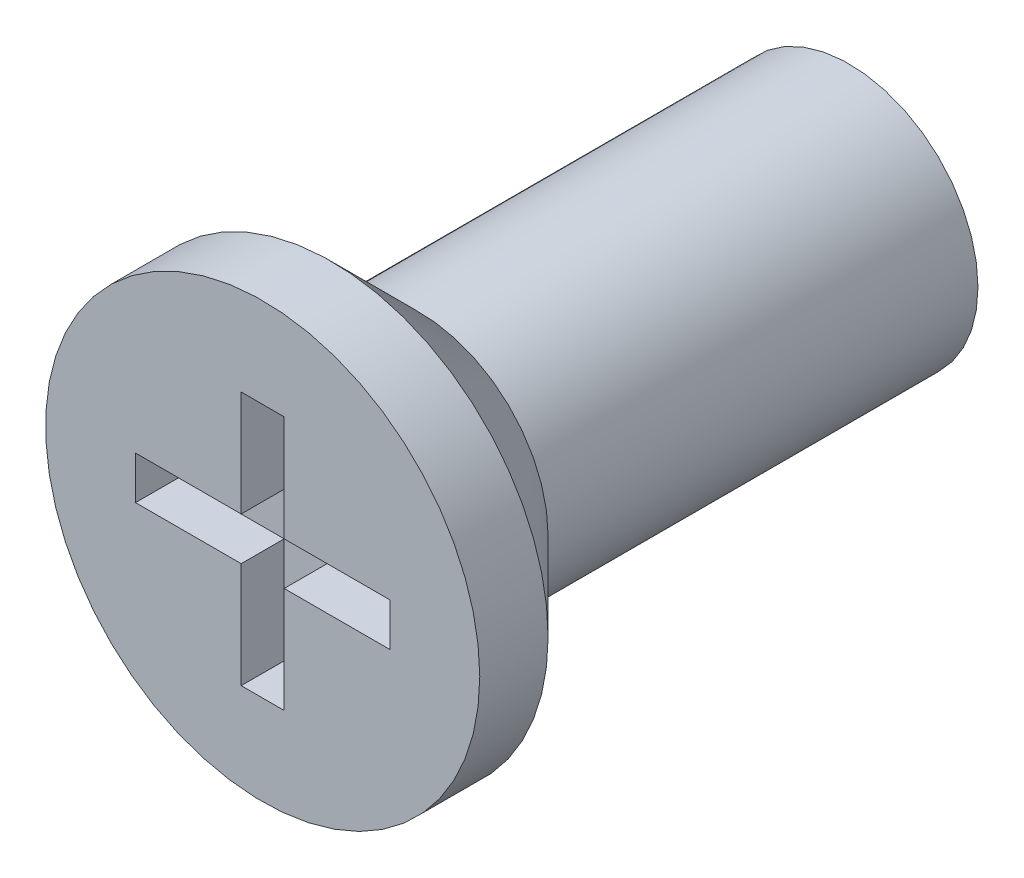
# Autodesk Inventor part: M3 Screw
Saved by Autodesk Inventor 2022.3 (Build 263350030, 350C)
## iProperties
Created: 2022-11-02
Part Number: M3 Screw
Material: Generic
Document SubType Name: Modeling
Designer: benka
Density: 1 g/cm^3
Appearance: Default
Author: benka
Autodesk Inventor part; units mm, degrees
ref_plane "YZ Plane" through (0, 0, 0) normal (1, 0, 0) x (0, 1, 0)
ref_plane "XZ Plane" through (0, 0, 0) normal (0, 1, 0) x (-1, 0, 0)
ref_plane "XY Plane" through (0, 0, 0) normal (0, 0, 1) x (1, 0, 0)
sketch "Sketch1" plane through (0, 0, 0) normal (0, 0, 1) x (1, 0, 0)
  circle A0 centre (-173.1851, -40.4973) radius 1.5
  point P0 (0, 0)
  dimension "d0" = 3
  constraints: 1 centre point
  measures "d0" diameter of A0
extrude "Extrusion1" add sketch "Sketch1" against normal blind 5
thread "Thread1" size "M3x0.5" class "6g" standard "ANSI Metric M Profile" full length
sketch "Sketch2" plane through (-173.1851, -40.4973, 0) normal (0, 0, 1) x (1, 0, 0)
  circle A0 centre (0, 0) radius 2.525
  point P0 (173.1851, 40.4973)
  dimension "d5" = 5.05
  constraints: 1 centre point, 1 coincident
  measures "d5" diameter of A0
extrude "Extrusion2" add sketch "Sketch2" along normal blind 1.82
ref_plane "Work Plane1" through (-173.1851, -40.4973, 1.32) normal (0, 0, 1) x (1, 0, 0)
chamfer "Chamfer1" distance 1.025 angle 45 1 edges at (-175.7101, -40.4973, 0)
sketch "Sketch3" plane through (-173.1851, -40.4973, 1.82) normal (0, 0, 1) x (1, 0, 0)
  line L0 (0, 1.5) -> (0, -1.5)
  line L1 (-1.5, 0) -> (1.5, 0)
  line L2 (-1.479, 0.25) -> (1.479, 0.25)
  line L3 (1.479, 0.25) -> (1.479, -0.25)
  line L4 (1.479, -0.25) -> (-1.479, -0.25)
  line L5 (-1.479, -0.25) -> (-1.479, 0.25)
  line L6 (-1.479, 0.25) -> (1.479, -0.25) construction
  line L7 (1.479, 0.25) -> (-1.479, -0.25) construction
  line L8 (0.25, 1.479) -> (-0.25, 1.479)
  line L9 (-0.25, 1.479) -> (-0.25, -1.479)
  line L10 (-0.25, -1.479) -> (0.25, -1.479)
  line L11 (0.25, -1.479) -> (0.25, 1.479)
  line L12 (0.25, 1.479) -> (-0.25, -1.479) construction
  line L13 (-0.25, 1.479) -> (0.25, -1.479) construction
  point P0 (173.1851, 40.4973)
  point P1 (0, 0)
  point P2 (-0.25, 0.25)
  point P3 (-0.25, -0.25)
  point P4 (0.25, -0.25)
  point P5 (0.25, 0.25)
  dimension "d12" = 0.5
  dimension "d13" = 0.5
  constraints: 28 end point, 4 midpoint, 4 parallel, 3 perpendicular, 2 horizontal, 1 vertical
  measures "d12" distance of L2.end L3.end
  measures "d13" distance of L10.end L9.end
extrude "Extrusion3" cut sketch "Sketch3" against normal blind 0.5
body "Solid1"
